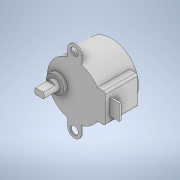
# Autodesk Inventor part: stepper-motor
Saved by Autodesk Inventor 2021 (Build 250183000, 183)
## iProperties
Created: 2024-04-22
Part Number: stepper-motor
Material: Generic
Document SubType Name: Modeling
Designer: Toby
Density: 1 g/cm^3
Appearance: Default
Author: Toby
Autodesk Inventor part; units mm, degrees
ref_plane "YZ Plane" through (0, 0, 0) normal (1, 0, 0) x (0, 1, 0)
ref_plane "XZ Plane" through (0, 0, 0) normal (0, 1, 0) x (-1, 0, 0)
ref_plane "XY Plane" through (0, 0, 0) normal (0, 0, 1) x (1, 0, 0)
sketch "Sketch1" plane through (0, 0, 0) normal (0, 0, 1) x (1, 0, 0)
  circle A0 centre (0, 0) radius 14
  dimension "d0" = 28
  constraints: 1 centre point, 1 coincident
  measures "d0" diameter of A0
extrude "Extrusion1" add sketch "Sketch1" along normal blind 19
sketch "Sketch2" plane through (0, 0, 19) normal (0, 0, 1) x (1, 0, 0)
  line L0 (10, 7.5) -> (16, 7.5)
  line L1 (16, 7.5) -> (16, -7.5)
  line L2 (16, -7.5) -> (10, -7.5)
  line L3 (10, -7.5) -> (10, 7.5)
  point P0 (0, 0)
  dimension "d3" = 15
  dimension "d4" = 10
  dimension "d5" = 16
  dimension "d6" = 7.5
  constraints: 8 end point, 2 parallel, 1 horizontal, 1 perpendicular
  measures "d3" distance of L0.end L1.end
  measures "d4" distance from line of point (0, 0) L3
  measures "d5" distance from line of L1 point (0, 0)
  measures "d6" distance from line of point (0, 0) L0
extrude "Extrusion2" add sketch "Sketch2" against normal blind 16.5
fillet "Fillet1" radius 1 2 edges at (16, 7.5, 10.75) (16, -7.5, 10.75)
sketch "Sketch3" plane through (0, 0, 19) normal (0, 0, 1) x (1, 0, 0)
  circle A0 centre (-8, 0) radius 4.5
  arc A1 (11.8216, 7.5) -> (11.8216, -7.5) centre (0, 0) ccw projected
  dimension "d10" = 9
  dimension "d11" = 0
  dimension "d12" = 8
  constraints: 1 centre point
  measures "d10" diameter of A0
  measures "d11" vertical distance of point (0, 0) A0.centre
  measures "d12" distance of A1.centre A0.centre
extrude "Extrusion3" add sketch "Sketch3" along normal blind 2
sketch "Sketch4" plane through (-8, 0, 21) normal (0, 0, 1) x (1, 0, 0)
  circle A0 centre (0, 0) radius 2.5
  point P0 (8, 0)
  dimension "d15" = 5
  constraints: 1 centre point
  measures "d15" diameter of A0
extrude "Extrusion4" add sketch "Sketch4" along normal blind 8
sketch "Sketch5" plane through (-8, 0, 29) normal (0, 0, 1) x (1, 0, 0)
  circle A0 centre (0, 0) radius 2.5 projected
  circle A1 centre (0, 0) radius 2.5
  line L0 (-3.3103, 1.5) -> (3.6339, 1.5)
  line L1 (3.6339, 1.5) -> (3.6339, -1.5)
  line L2 (3.6339, -1.5) -> (-3.3103, -1.5)
  line L3 (-3.3103, -1.5) -> (-3.3103, 1.5)
  point P0 (8, 0)
  point P1 (2, -1.5)
  point P2 (-2, -1.5)
  point P3 (-2, 1.5)
  point P4 (2, 1.5)
  dimension "d18" = 3
  dimension "d19" = 1.5
  constraints: 8 end point, 2 parallel, 1 centre point, 1 coincident, 1 horizontal, 1 perpendicular
  measures "d18" distance of L2.end L0.start
  measures "d19" distance from line of A1.centre L0
extrude "Extrusion5" cut sketch "Sketch5" against normal blind 6 contours L0 A0 | A0 L2
sketch "Sketch6" plane through (16, -6.5, 19) normal (1, 0, 0) x (0, 0, -1)
  line L0 (2, 10.5) -> (3, 10.5)
  line L1 (3, 10.5) -> (3, 2.5)
  line L2 (3, 2.5) -> (2, 2.5)
  line L3 (2, 2.5) -> (2, 10.5)
  line L4 (0, 0) -> (0, 13) projected
  line L5 (16.5, 14) -> (0, 14) projected
  line L6 (0, -1) -> (16.5, -1) projected
  point P0 (19, 6.5)
  dimension "d22" = 2
  dimension "d23" = 1
  dimension "d24" = 3.5
  dimension "d25" = 3.5
  constraints: 8 end point, 2 parallel, 1 horizontal, 1 perpendicular
  measures "d22" distance between parallel lines of L4 L3
  measures "d23" distance between parallel lines of L1 L3
  measures "d24" distance between parallel lines of L0 L5
  measures "d25" distance between parallel lines of L6 L2
extrude "Extrusion6" add sketch "Sketch6" along normal blind 5
sketch "Sketch7" plane through (0, 0, 19) normal (0, 0, 1) x (1, 0, 0)
  line L0 (-3.5, 12) -> (3.5, 12)
  line L1 (3.5, 12) -> (3.5, 21)
  line L2 (3.5, 21) -> (-3.5, 21)
  line L3 (-3.5, 21) -> (-3.5, 12)
  arc A0 (11.8216, 7.5) -> (11.8216, -7.5) centre (0, 0) ccw projected
  line L4 (-3.5, -12) -> (3.5, -12)
  line L5 (3.5, -12) -> (3.5, -21)
  line L6 (3.5, -21) -> (-3.5, -21)
  line L7 (-3.5, -21) -> (-3.5, -12)
  point P0 (0, 14)
  point P1 (0, -14)
  point P2 (3.5, -13.5554)
  point P3 (-3.5, -13.5554)
  point P4 (-3.5, 13.5554)
  point P5 (3.5, 13.5554)
  dimension "d28" = 7
  dimension "d29" = 7
  dimension "d30" = 3.5
  dimension "d31" = 2
  dimension "d32" = 7
  dimension "d33" = 7
  dimension "d34" = 2
  dimension "d35" = 3.5
  constraints: 16 end point, 4 parallel, 2 horizontal, 2 perpendicular, 2 point on circle
  measures "d28" distance from line of point (0, 14) L2
  measures "d29" distance of L1.end L2.end
  measures "d30" distance from line of point (0, 0) L3
  measures "d31" distance from line of point (0, 14) L0
  measures "d32" distance of L5.end L6.end
  measures "d33" distance from line of L6 point (0, -14)
  measures "d34" distance from line of point (0, -14) L4
  measures "d35" distance from line of point (0, -14) L7
extrude "Extrusion7" add sketch "Sketch7" against normal blind 0.5 contours A0 L5 L6 L7 | L3 L2 L1 A0
fillet "Fillet2" radius 3.5 4 edges at (-3.5, 21, 18.75) (3.5, 21, 18.75) (-3.5, -21, 18.75) (3.5, -21, 18.75)
sketch "Sketch8" plane through (0, 0, 19) normal (0, 0, 1) x (1, 0, 0)
  arc A0 (3.5, 17.5) -> (-3.5, 17.5) centre (0, 17.5) ccw projected
  arc A1 (-3.5, -17.5) -> (3.5, -17.5) centre (0, -17.5) ccw projected
  point P0 (0, 0)
  dimension "d39" = 0
  constraints: 1 coincident
  measures "d39" distance of A0.centre point (0, 17.5)
hole "Hole1" at (0, 17.5, 19) at (0, -17.5, 19) direction (0, 0, -1) diameter 4 depth 1 tip angle 118
body "Solid1"
